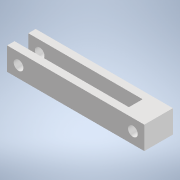
# Autodesk Inventor part: connectiingRodV03
Saved by Autodesk Inventor 2020.2 (Build 242310000, 310)
## iProperties
Created: 2020-01-21
Part Number: connectiingRodV03
Material: Generic
Document SubType Name: Modeling
Designer: robst
Density: 1 g/cm^3
Appearance: Default
Author: robst
Autodesk Inventor part; units mm, degrees
ref_plane "YZ Plane" through (0, 0, 0) normal (1, 0, 0) x (0, 1, 0)
ref_plane "XZ Plane" through (0, 0, 0) normal (0, 1, 0) x (-1, 0, 0)
ref_plane "XY Plane" through (0, 0, 0) normal (0, 0, 1) x (1, 0, 0)
sketch "Sketch1" plane through (0, 0, 0) normal (0, 0, 1) x (1, 0, 0)
  line L0 (0, 0) -> (165.1, 0)
  line L1 (165.1, 0) -> (165.1, 12.7)
  line L2 (165.1, 12.7) -> (0, 12.7)
  line L3 (0, 12.7) -> (0, 0)
  line L4 (165.1, 0) -> (165.1, -12.7)
  line L5 (165.1, -12.7) -> (0, -12.7)
  line L6 (0, -12.7) -> (0, 0)
  dimension "d2" = 165.1
  dimension "d3" = 25.4
  constraints: 14 end point, 2 parallel, 2 symmetric about line, 1 horizontal, 1 perpendicular
  measures "d2" distance of L1.end L2.end
  measures "d3" distance between parallel lines of L5 L2
extrude "Extrusion1" add sketch "Sketch1" along normal mid plane 31.75
sketch "Sketch3" plane through (0, 12.7, 15.875) normal (0, 1, 0) x (1, 0, 0)
  line L0 (0, 15.875) -> (165.1, 15.875) construction
  line L1 (165.1, 31.75) -> (165.1, 0) construction
  line L2 (0, 31.75) -> (0, 0) projected
  line L3 (0, 23.495) -> (139.7, 23.495)
  line L4 (139.7, 23.495) -> (139.7, 15.875)
  line L5 (0, 23.495) -> (0, 15.875)
  line L6 (0, 0) -> (0, 31.75)
  line L7 (0, 8.255) -> (139.7, 8.255)
  line L8 (139.7, 8.255) -> (139.7, 15.875)
  dimension "d6" = 139.7
  dimension "d7" = 7.62
  constraints: 14 end point, 4 symmetric about line, 3 point on line, 1 collinear, 1 horizontal, 1 midpoint, 1 perpendicular
  measures "d6" distance of L3.start L3.end
  measures "d7" distance of L3.end L4.end
extrude "Extrusion2" cut sketch "Sketch3" against normal through all
sketch "Sketch4" plane through (0, 0, 15.875) normal (0, 0, 1) x (1, 0, 0)
  circle A0 centre (12.7, 0) radius 5.3975
  circle A1 centre (152.4, 0) radius 5.3975
  line L0 (165.1, -12.7) -> (165.1, 12.7) projected
  point P0 (0, 0)
  dimension "d10" = 10.795
  dimension "d11" = 12.7
  dimension "d12" = 12.7
  constraints: 2 centre point, 1 equal radius
  measures "d10" diameter of A0
  measures "d11" distance of A0.centre point (0, 0)
  measures "d12" distance from line of A1.centre L0
extrude "Extrusion3" cut sketch "Sketch4" against normal through all
body "Solid1"
